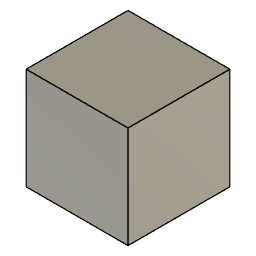
Day1_Cube (Autodesk Fusion 360 design; units mm, degrees)
part number: 2025-10-10-20-38-47-019
part number: 2025-10-10-20-43-26-079
part number: 2025-10-10-20-46-29-798
Autodesk Fusion 360 part; units mm, degrees
sketch "Sketch1" plane through (0, 0, 0) normal (0, 0, 1) x (1, 0, 0) in component "Box"
  line L0 (41.5, 17) -> (-41.5, 17)
  line L1 (-41.5, 17) -> (-41.5, -17)
  line L2 (-41.5, -17) -> (41.5, -17)
  line L3 (41.5, -17) -> (41.5, 17)
  line L4 (41.5, 17) -> (-41.5, -17) construction
  line L5 (-41.5, 17) -> (41.5, -17) construction
  dimension "d1" = 83
  dimension "d2" = 34
  constraint horizontal L0
  constraint perpendicular L0 L1
  constraint parallel L0 L2
  constraint parallel L1 L3
  constraint coincident L4 origin
  constraint coincident L5 origin
  measures "d1" distance of L1.end L2.end
  measures "d2" distance of L0.end L1.end
sketch "Sketch3" plane through (0, 0, 0) normal (0, 0, 1) x (1, 0, 0) in component "Box"
  line L0 (9.6543, -10) -> (-10.3457, -10)
  line L1 (-10.3457, -10) -> (-10.3457, 10)
  line L2 (-10.3457, 10) -> (9.6543, 10)
  line L3 (9.6543, 10) -> (9.6543, -10)
  line L4 (9.6543, -10) -> (-10.3457, 10) construction
  line L5 (-10.3457, -10) -> (9.6543, 10) construction
  point P0 (-0.3457, 0)
  dimension "d14" = 20
  constraint horizontal L0
  constraint perpendicular L0 L1
  constraint parallel L0 L2
  constraint parallel L1 L3
  constraint coincident L4 P0
  constraint coincident L5 P0
  measures "d14" distance of L1.end L2.end
extrude "Extrude3" add sketch "Sketch3" along normal blind 20 in component "Box"
component "Lid" placed x (1, 0, 0) y (0, 1, 0) z (0, 0, 1) at (0, 0, 0)
component "Box" placed x (1, 0, 0) y (0, 1, 0) z (0, 0, 1) at (0, 0, 0) in component "Lid"
